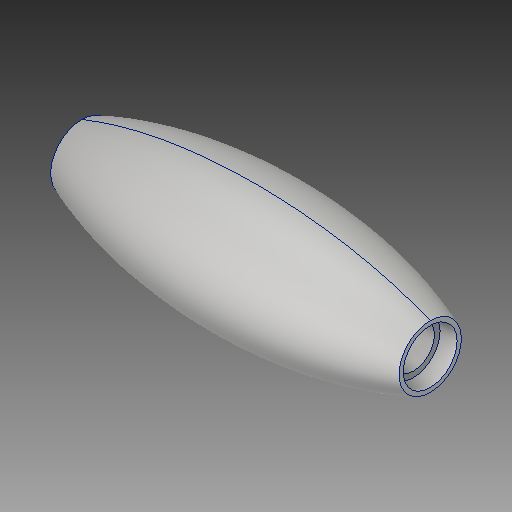
# Autodesk Inventor part: roller 8-19-6 bearing
Saved by Autodesk Inventor 2018 (Build 220112000, 112)
## iProperties
Created: 2017-08-22
Part Number: roller 8-19-6 bearing
Material: Aluminum 6061
Document SubType Name: Modeling
Designer: P445885
Density: 2.7 g/cm^3
Appearance: Aluminum - Flat
Mass: 306.459 g
Surface Area: 209.296 cm^2
Volume: 113.503 cm^3
Author: P445885
Autodesk Inventor part; units mm, degrees
ref_plane "YZ Plane" through (0, 0, 0) normal (1, 0, 0) x (0, 1, 0)
ref_plane "XZ Plane" through (0, 0, 0) normal (0, 1, 0) x (-1, 0, 0)
ref_plane "Work Plane1" through (0, 0, 0) normal (0, -0.8660254, 0.5) x (1, 0, 0)
sketch "Sketch1" plane through (0, 0, 0) normal (0, -0.8660254, 0.5) x (1, 0, 0)
  circle A0 centre (0, 0) radius 97 construction
  dimension "d1" = 194
  constraints: 1 centre point, 1 coincident
  measures "d1" diameter of A0
sketch "Sketch2" plane through (0, 0, 0) normal (0, 0, 1) x (1, 0, 0)
  circle A0 centre (0, 26.5) radius 22 construction
  ellipse E0 centre (0, 0) end of major axis (97, 0) minor radius 48.5 construction
  line L0 (0, 26.5) -> (-61.5142, 26.5)
  line L1 (0, 37.5) -> (-61.5142, 37.5) construction
  line L2 (-61.5142, 37.5) -> (-61.5142, 26.5)
  line L3 (0, 0) -> (0, 48.5) construction
  line L4 (0, 26.5) -> (61.5142, 26.5)
  line L5 (61.5142, 37.5) -> (61.5142, 26.5)
  ellipse E1 centre (0, 0) end of major axis (97, 0) minor radius 48.5 (61.5142, 37.5) -> (-61.5142, 37.5) ccw
  dimension "d2" = 44
  dimension "d3" = 11
  constraints: 13 end point, 2 symmetric about line, 2 vertical alignment, 1 coincident, 1 horizontal, 1 parallel, 1 perpendicular, 9 other
  measures "d3" distance between parallel lines of L0 L1
revolve "Revolution1" add sketch "Sketch2" angle 360 about axis through (0, 26.5, 0) along (1, 0, 0)
sketch "Sketch3" plane through (61.5142, 26.5, 0) normal (1, 0, 0) x (0, 0, -1)
  circle A0 centre (0, 0) radius 11 projected
  circle A1 centre (0, 0) radius 9.5
  point P0 (0, -26.5)
  point P1 (0, 11)
  dimension "d5" = 19
  constraints: 1 centre point, 1 coincident, 1 vertical alignment
  measures "d5" diameter of A1
extrude "Extrusion1" cut sketch "Sketch3" against normal blind 6 contours A1
sketch "Sketch4" plane through (-61.5142, 26.5, 0) normal (-1, 0, 0) x (0, 0, 1)
  circle A0 centre (0, 0) radius 9.5
  dimension "d8" = 19
  constraints: 1 centre point
  measures "d8" diameter of A0
extrude "Extrusion2" cut sketch "Sketch4" against normal blind 6
hole "Hole1" at (-55.5142, 26.5, 0) direction (1, 0, 0) diameter 15 end up to face face through (55.5142, 28.5999, -1.6069) facing (1, 0, 0)
body "Solid1"
